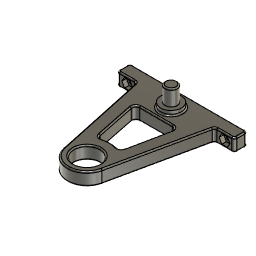
Spring Frame Front v5 (Autodesk Fusion 360 design; units mm, degrees)
Autodesk Fusion 360 part; units mm, degrees
sketch "base" plane through (0, 0, 0) normal (0, 0, 1) x (1, 0, 0)
  line L0 (-43.1936, 36.1554) -> (-0.1936, 36.1554)
  line L1 (-45.1936, 28.1554) -> (-45.1936, 34.1554)
  arc A0 (-43.1936, 36.1554) -> (-45.1936, 34.1554) centre (-43.1936, 34.1554) ccw
  arc A1 (-45.1936, 28.1554) -> (-43.1936, 26.1554) centre (-43.1936, 28.1554) ccw
  line L2 (-43.1936, 26.1554) -> (-31.8136, 26.1554)
  line L3 (-0.1936, 36.1554) -> (-0.1936, -56.8446) construction
  circle A2 centre (-0.1936, -41.8446) radius 15
  arc A3 (-29.8585, 24.5769) -> (-31.8136, 26.1554) centre (-31.8136, 24.1554) ccw
  arc A4 (16.5665, -35.2796) -> (-16.9537, -35.2796) centre (-0.1936, -41.8446) ccw
  line L4 (-14.8567, -45.006) -> (-29.8585, 24.5769)
  line L5 (-0.1936, 36.1554) -> (-0.1936, 11.1554) construction
  line L6 (-0.1936, 11.1554) -> (-12.6936, 11.1554)
  line L7 (-15.6324, 7.5526) -> (-9.3579, -23.0377)
  arc A5 (-12.6936, 11.1554) -> (-15.6324, 7.5526) centre (-12.6936, 8.1554) ccw
  arc A6 (-9.4825, -22.4305) -> (-5.6365, -24.6873) centre (-6.5436, -21.8277) ccw
  line L8 (-31.8136, 26.1554) -> (-43.1936, 26.1554)
  arc A7 (44.8064, 34.1554) -> (42.8064, 36.1554) centre (42.8064, 34.1554) ccw
  line L9 (44.8064, 28.1554) -> (44.8064, 34.1554)
  line L10 (15.2452, 7.5526) -> (8.9707, -23.0377)
  line L11 (42.8064, 26.1554) -> (31.4264, 26.1554)
  arc A8 (15.2452, 7.5526) -> (12.3064, 11.1554) centre (12.3064, 8.1554) ccw
  arc A9 (31.4264, 26.1554) -> (29.4713, 24.5769) centre (31.4264, 24.1554) ccw
  line L12 (31.4264, 26.1554) -> (42.8064, 26.1554)
  line L13 (-0.1936, 11.1554) -> (12.3064, 11.1554)
  line L14 (42.8064, 36.1554) -> (-0.1936, 36.1554)
  arc A10 (42.8064, 26.1554) -> (44.8064, 28.1554) centre (42.8064, 28.1554) ccw
  line L15 (14.4695, -45.006) -> (29.4713, 24.5769)
  arc A11 (5.2493, -24.6873) -> (9.0953, -22.4305) centre (6.1564, -21.8277) ccw
  circle A12 centre (-0.1936, -41.8446) radius 10
  line L16 (-0.1936, 36.1554) -> (-0.1936, 22.6554) construction
  circle A13 centre (-0.1936, 22.6554) radius 8
  circle A14 centre (-0.1936, 22.6554) radius 4.7
  point P0 (-45.1936, 36.1554)
  point P1 (44.8064, 36.1554)
  point P2 (-45.1936, 26.1554)
  point P3 (44.8064, 26.1554)
  point P4 (44.8064, 36.1554)
  dimension "d1" = 90
  dimension "d2" = 10
  dimension "d3" = 2
  dimension "d4" = 11.38
  dimension "d5" = 93
  dimension "d6" = 4
  dimension "d7" = 30
  dimension "d8" = 36
  dimension "d9" = 25
  dimension "d10" = 12.5
  dimension "d11" = 6
  dimension "d12" = 6
  dimension "d13" = 20
  dimension "d16" = 13.5
  dimension "d17" = 16
  dimension "d18" = 9.4
  constraint horizontal L0
  constraint vertical L1
  constraint coincident P0 L0
  constraint coincident P0 L1
  constraint tangent L0 A0
  constraint tangent L1 A0
  constraint coincident P2 L1
  constraint tangent L1 A1
  constraint equal A0 A1
  constraint coincident P4 L0
  constraint vertical L2.end A3.centre
  constraint coincident L3 A2.centre
  constraint coincident L3.end A2
  constraint concentric A2 A4
  constraint coincident A2 L4.start
  constraint perpendicular L5 L6
  constraint tangent L6 A5
  constraint vertical L6.end A5.centre
  constraint tangent A4 A6
  constraint tangent L7 A6
  constraint tangent L7 A5
  constraint coincident A4 A6.end
  constraint coincident L7 A6.start
  constraint symmetric P0 L3 P4
  constraint symmetric P2 L3 P3
  constraint symmetric L0.start L3 A7.end
  constraint symmetric L1.end L3 A7.start
  constraint symmetric A0 L3 A7
  constraint symmetric L1.start L3 L9.start
  constraint symmetric A1.end L3 L11.start
  constraint symmetric A1 L3 A10
  constraint symmetric L2.end L3 L11.end
  constraint symmetric L0.end L3 L5.start
  constraint symmetric L3 A3.start A9.end
  constraint symmetric L3 A3 A9
  constraint symmetric L3 A4.end A4.start
  constraint symmetric L3 L4.start L15.start
  constraint symmetric L3 L5.end L6.start
  constraint symmetric L3 L6.end A8.end
  constraint symmetric L3 L7.end L10.end
  constraint symmetric L3 L7.start L10.start
  constraint symmetric L3 A5 A8
  constraint symmetric L3 A6.end A11.start
  constraint symmetric L3 A6.start A11.end
  constraint symmetric L3 A6 A11
  constraint concentric A4 A12
  constraint coincident L5 L16.end
  constraint coincident L3 L16.end
  constraint coincident L16.end A13.centre
  measures "d1" distance of P0 P4
  measures "d2" distance of P0 P2
  measures "d3" radius of A0
  measures "d4" distance of A1.end L2.end
  measures "d5" distance of L0.end L3.end
  measures "d6" diameter of A3
  measures "d7" diameter of A2
  measures "d8" diameter of A4
  measures "d9" distance of L0.end L5.end
  measures "d10" distance of L5.end L6.end
  measures "d11" diameter of A5
  measures "d12" diameter of A6
  measures "d13" diameter of A12
  measures "d16" distance of L0.end L16.end
  measures "d17" diameter of A13
  measures "d18" diameter of A14
extrude "Extrude1" add sketch "base" along normal blind 10 contours L0 L1 A0 A1 L2 A3 A4 L4 L6 L7 A5 A6 L8 A7 L9 L10 L11 A8 A9 L12 L13 L14 A10 L15 A11 | A2 A4 L4 L15 | A2 | A13 | A14
extrude "Extrude2" add sketch "base" along normal blind 13.5 contours A13
extrude "Extrude3" add sketch "base" along normal blind 25.5 contours A14
fillet "Fillet1" radius 1 24 edges at (-0.1936, 11.1554, 10) (14.6311, 10.0516, 10) (12.1702, -7.439, 10) (7.6747, -24.4152, 10) (-0.1936, -23.8446, 10) (-8.0619, -24.4152, 10) (-12.5574, -7.439, 10) (-15.0183, 10.0516, 10) (21.9704, -10.2145, 10) (30.17, 25.7115, 10) (37.1164, 26.1554, 10) (44.2206, 26.7411, 10) (44.8064, 31.1554, 10) (44.2206, 35.5696, 10) (-0.1936, 36.1554, 10) (-44.6078, 35.5696, 10) (-45.1936, 31.1554, 10) (-44.6078, 26.7411, 10) (-37.5036, 26.1554, 10) (-30.5572, 25.7115, 10) (-22.3576, -10.2145, 10) (-0.1936, -56.8446, 10) (-9.5169, -38.2285, 10) (-4.5755, 20.9558, 25.5)
fillet "Fillet1" radius 1 23 edges at (30.17, 25.7115, 0) (37.1164, 26.1554, 0) (44.2206, 26.7411, 0) (44.8064, 31.1554, 0) (44.2206, 35.5696, 0) (-0.1936, 36.1554, 0) (-44.6078, 35.5696, 0) (-45.1936, 31.1554, 0) (-44.6078, 26.7411, 0) (-37.5036, 26.1554, 0) (-30.5572, 25.7115, 0) (-22.3576, -10.2145, 0) (-0.1936, -56.8446, 0) (21.9704, -10.2145, 0) (12.1702, -7.439, 0) (7.6747, -24.4152, 0) (-0.1936, -23.8446, 0) (-8.0619, -24.4152, 0) (-12.5574, -7.439, 0) (-15.0183, 10.0516, 0) (-0.1936, 11.1554, 0) (14.6311, 10.0516, 0) (-9.5169, -38.2285, 0)
fillet "Fillet2" radius 1 1 edges at (-7.6522, 25.5483, 10)
sketch "holes" plane through (0, 26.1554, 0) normal (0, -1, 0) x (1, 0, 0)
  line L0 (31.4264, 1) -> (42.8064, 1)
  line L1 (42.8064, 1) -> (42.8064, 9)
  line L2 (42.8064, 9) -> (31.4264, 9)
  line L3 (31.4264, 9) -> (31.4264, 1)
  line L4 (42.8064, 5) -> (37.3064, 5) construction
  circle A0 centre (37.3064, 5) radius 2.2
  line L5 (41.4564, 5) -> (39.3814, 8.594)
  line L6 (39.3814, 8.594) -> (35.2314, 8.594)
  line L7 (35.2314, 8.594) -> (33.1564, 5)
  line L8 (33.1564, 5) -> (35.2314, 1.406)
  line L9 (35.2314, 1.406) -> (39.3814, 1.406)
  line L10 (39.3814, 1.406) -> (41.4564, 5)
  line L11 (0, 20) -> (0, 2.5) construction
  line L12 (-41.4564, 5) -> (-39.3814, 8.594)
  line L13 (-39.3814, 8.594) -> (-35.2314, 8.594)
  line L14 (-35.2314, 8.594) -> (-33.1564, 5)
  line L15 (-33.1564, 5) -> (-35.2314, 1.406)
  line L16 (-35.2314, 1.406) -> (-39.3814, 1.406)
  circle A1 centre (-37.3064, 5) radius 2.2
  line L17 (-39.3814, 1.406) -> (-41.4564, 5)
  point P0 (37.3064, 5)
  dimension "d26" = 5.5
  dimension "d27" = 4.4
  dimension "d28" = 4.15
  constraint midpoint L1 L4.start
  constraint perpendicular L1 L4
  constraint coincident P0 L4.end
  constraint coincident L4 L5.start
  constraint symmetric A0 L11 A1
  constraint symmetric L5.start L11 L12.start
  constraint symmetric L5.end L11 L12.end
  constraint symmetric L6.end L11 L13.end
  constraint symmetric L7.end L11 L14.end
  constraint symmetric L8.end L11 L15.end
  constraint symmetric L9.end L11 L16.end
  measures "d26" distance of L4.start P0
  measures "d27" diameter of A0
  measures "d28" distance of L5.start P0
extrude "Extrude4" cut sketch "holes" against normal blind 21 contours A0
extrude "Extrude5" cut sketch "holes" against normal blind 3.5 contours L5 L6 L7 L8 L9 L10
extrude "Extrude6" cut sketch "holes" against normal blind 14 contours A1
extrude "Extrude7" cut sketch "holes" against normal blind 3.5 contours L12 L13 L14 L15 L16 L17
named bodies: "SpringFrameFront"
